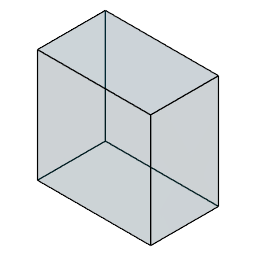
Cristal 6mm (Autodesk Fusion 360 design; units mm, degrees)
part number: 2025-12-28-18-55-12-011
Autodesk Fusion 360 part; units mm, degrees
sketch "Boceto1" plane through (0, 0, 0) normal (1, 0, 0) x (0, 1, 0)
  line L0 (0, 0) -> (6, 0)
  line L1 (6, 0) -> (6, 10)
  line L2 (6, 10) -> (0, 10)
  line L3 (0, 10) -> (0, 0)
  dimension "d2" = 10
  dimension "d3" = 6
  constraint horizontal L0
  constraint vertical L1
  constraint horizontal L2
  constraint vertical L3
  constraint coincident L0.start L3.end
  measures "d2" distance of L0.start L2.end
  measures "d3" distance of L0.start L0.end
extrude "Extruir1" add sketch "Boceto1" along normal blind 10
equation "L = 10 mm"
equation "d2 = L"
equation "d4 = L"
